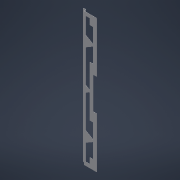
# Autodesk Inventor part: SP56V1 Chapa Detectores
Saved by Autodesk Inventor 2021.2 (Build 252289000, 289)
## iProperties
Created: 2026-10-05
Part Number: SP56V1 Chapa Detectores
Material: Steel, Carbon
Document SubType Name: Sheet Metal
Designer: nelso
Density: 7.87 g/cm^3
Sheet Metal Rule: DD 1.56mm
Appearance: White
Mass: 1429.19 g
Surface Area: 2406.13 cm^2
Volume: 181.6 cm^3
Author: nelso
Autodesk Inventor part; units mm, degrees
ref_plane "YZ Plane" through (0, 0, 0) normal (1, 0, 0) x (0, 1, 0)
ref_plane "XZ Plane" through (0, 0, 0) normal (0, 1, 0) x (-1, 0, 0)
ref_plane "XY Plane" through (0, 0, 0) normal (0, 0, 1) x (1, 0, 0)
sketch "Sketch1" plane through (0, 0, 0) normal (0, 1, 0) x (-1, 0, 0)
  line L0 (-30, 565) -> (30, 565) construction
  line L1 (30, 565) -> (30, -565) construction
  line L2 (30, -565) -> (-30, -565) construction
  line L3 (-30, -565) -> (-30, 565) construction
  line L4 (-30, 565) -> (30, -565) construction
  line L5 (30, 565) -> (-30, -565) construction
  line L6 (30, -565) -> (0, -565)
  line L7 (0, -565) -> (0, -485)
  line L8 (0, -485) -> (30, -485)
  line L9 (30, -485) -> (30, -565)
  line L10 (-30, -565) -> (0, -565)
  line L11 (0, -565) -> (0, -135)
  line L12 (0, -135) -> (-30, -135)
  line L13 (-30, -135) -> (-30, -565)
  line L14 (30, -135) -> (30, -215)
  line L15 (30, -215) -> (0, -215)
  line L16 (0, -215) -> (0, 215)
  line L17 (0, 215) -> (30, 215)
  line L18 (30, 215) -> (30, -215)
  line L19 (-30, 565) -> (0, 565)
  line L20 (0, 565) -> (0, 135)
  line L21 (0, 135) -> (-30, 135)
  line L22 (-30, 135) -> (-30, 565)
  line L23 (30, 565) -> (0, 565)
  line L24 (0, 565) -> (0, 485)
  line L25 (0, 485) -> (30, 485)
  line L26 (30, 485) -> (30, 565)
  point P0 (0, 0)
  dimension "d0" = 60
  dimension "d1" = 1130
  dimension "d2" = 80
  dimension "d3" = 430
  dimension "d4" = 80
  dimension "d5" = 430
  dimension "d6" = 430
  dimension "d7" = 80
  measures "d0" distance of L1.end L2.end
  measures "d1" distance of L0.end L1.end
  measures "d2" distance of L6.end L7.end
  measures "d3" distance of L11.end L10.end
  measures "d4" distance of L14.start L14.end
  measures "d5" distance of L15.end L16.end
  measures "d6" distance of L19.end L20.end
  measures "d7" distance of L24.end L23.end
extrude "Plate1" add sketch "Sketch1" along normal blind 1.56
sketch "Sketch2" plane through (0, 0, 0) normal (0, -1, 0) x (1, 0, 0)
  line L0 (-30, 485) -> (-30, 565)
  line L1 (-30, 565) -> (-80, 565)
  line L2 (-80, 565) -> (-80, 535)
  line L3 (-80, 535) -> (-30, 535)
  line L4 (-30, 535) -> (-30, 565)
  line L5 (-30, -485) -> (-30, -565)
  line L6 (-30, -565) -> (-80, -565)
  line L7 (-80, -565) -> (-80, -535)
  line L8 (-80, -535) -> (-30, -535)
  line L9 (-30, -535) -> (-30, -565)
  line L10 (-80, 565) -> (-80, -565)
  line L11 (0, 485) -> (0, 215)
  line L12 (-30, 215) -> (-30, -215)
  line L13 (-30, 0) -> (-15, 0)
  line L14 (0, -485) -> (0, -215)
  line L15 (0, -350) -> (15, -350)
  line L16 (-15, 0) -> (-80, -37.5278)
  line L17 (-80, 37.5278) -> (-15, 0)
  line L18 (-80, -565) -> (-65, -565)
  line L19 (-65, -565) -> (-65, 565)
  line L20 (-65, 565) -> (-80, 565)
  line L21 (-80, 565) -> (-80, -565)
  line L22 (0, 350) -> (15, 350)
  line L23 (15, 350) -> (-80, 295.1517)
  line L24 (-80, 404.8483) -> (15, 350)
  line L25 (-30, 565) -> (-80, 565)
  line L26 (-80, 565) -> (-80, 535)
  line L27 (-80, 535) -> (-30, 535)
  line L28 (-30, 535) -> (-30, 565)
  line L29 (15, -350) -> (-80, -404.8483)
  line L30 (-80, -295.1517) -> (15, -350)
  point P0 (0, 0)
  point P1 (-80, 0)
  point P2 (-80, 350)
  point P3 (-80, -350)
  dimension "d9" = 50
  dimension "d10" = 30
  dimension "d11" = 50
  dimension "d12" = 30
  dimension "d14" = 15
  dimension "d15" = 15
  dimension "d16" = 15
  measures "d9" distance of L3.end L2.end
  measures "d10" distance of L2.end L1.end
  measures "d11" distance of L7.end L8.end
  measures "d12" distance of L6.end L7.end
  measures "d14" distance of L13.start L13.end
  measures "d15" distance of L15.start L15.end
  measures "d16" distance of L20.end L19.end
sheet face with bend "Face2" sketch "Sketch2" thickness 1.56 toward (0, 1, 0) bend radius 1.212
bend "Bend1"
sketch "Sketch3" plane through (-78.44, 0, 565) normal (-1, 0, 0) x (0, -1, 0)
  line L0 (0, -1130) -> (0, 0)
  line L1 (0, 0) -> (-20, 0)
  line L2 (-20, 0) -> (-20, -1130)
  line L3 (-20, -1130) -> (0, -1130)
  constraints: 6 end point, 1 horizontal, 1 perpendicular, 1 vertical
edge flange "Flange1" height 20 angle 90 thickness 1.56 bend radius 1.212 thickness toward (-1, 0, 0) relief tear relief width 1.56 relief depth 0.78 edges at (-80, 1.56, 0) wall of the first edge with corners at (-78.44, 0, -565) (-78.44, 0, 565) (-78.44, 20, 565) (-78.44, 20, -565)
bend "Bend2"
corner "Corner1"
sketch "Sketch4" plane through (-78.44, 18.44, -565) normal (0, 1, 0) x (-1, 0, 0)
  line L0 (0, 1130) -> (0, 0)
  line L1 (0, 0) -> (25, 0)
  line L2 (25, 0) -> (25, 1130)
  line L3 (25, 1130) -> (0, 1130)
  constraints: 6 end point, 1 horizontal, 1 perpendicular, 1 vertical
edge flange "Flange2" height 25 angle 90 thickness 1.56 bend radius 1.212 thickness toward (0, 1, 0) relief tear relief width 1.56 relief depth 0.78 edges at (-80, 20, 0) wall of the first edge with corners at (-78.44, 18.44, 565) (-78.44, 18.44, -565) (-103.44, 18.44, -565) (-103.44, 18.44, 565)
bend "Bend3"
corner "Corner2"
fillet "Corner Round1" radius 3 24 edges at (-30, 0.78, 485) (30, 0.78, 565) (-30, 0.78, 215) (30, 0.78, 135) (-30, 0.78, 8.6603) (-65, 0.78, 28.8675) (-30, 0.78, -8.6603) (-65, 0.78, -28.8675) (30, 0.78, -135) (-30, 0.78, -215) (-30, 0.78, -485) (-65, 0.78, -535) (30, 0.78, -565) (-103.44, 19.22, 565) (0, 0.78, 358.6603) (0, 0.78, 341.3397) (-65, 0.78, 396.188) (-65, 0.78, 303.812) (0, 0.78, -341.3397) (0, 0.78, -358.6603) (-65, 0.78, -303.812) (-65, 0.78, -396.188) (-103.44, 19.22, -565) (-65, 0.78, 535)
equation "\"d8\" = Thickness"
equation "\"d17\" = BendRadius"
equation "\"d18\" = BendReliefWidth"
equation "\"d20\" = MinimumRemnant"
equation "\"d19\" = BendReliefDepth"
equation "\"d21\" = TransitionRadius"
equation "\"d22\" = BendReliefWidth"
equation "\"d23\" = BendReliefDepth"
equation "\"d24\" = MinimumRemnant"
equation "\"d25\" = TransitionRadius"
equation "\"d28\" = BendRadius"
equation "\"d29\" = CornerReliefSize"
equation "\"d30\" = GapSize"
equation "\"d31\" = JacobiRadiusSize"
equation "\"d32\" = BendReliefWidth"
equation "\"d33\" = BendReliefDepth"
equation "\"d34\" = MinimumRemnant"
equation "\"d35\" = TransitionRadius"
equation "\"d38\" = BendRadius"
equation "\"d39\" = CornerReliefSize"
equation "\"d40\" = GapSize"
equation "\"d41\" = JacobiRadiusSize"
equation "\"BendReliefWidth\" = Thickness"
equation "\"BendReliefDepth\" = 0.5 * Thickness"
equation "\"CornerReliefSize\" = 4 * Thickness"
equation "\"MinimumRemnant\" = 2 * Thickness"
equation "\"TransitionRadius\" = BendRadius"
equation "\"JacobiRadiusSize\" = BendRadius"
equation "\"GapSize\" = Thickness"
equation "\"Thickness\" = 1.56"
equation "\"BendRadius\" = 1.212"
body "Solid1"
